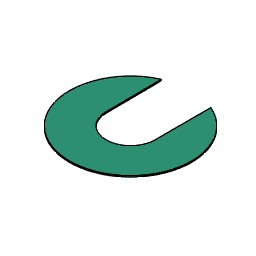
0.2 mm slidable washer - 8mm Shaft v1 (Autodesk Fusion 360 design; units mm, degrees)
Autodesk Fusion 360 part; units mm, degrees
note: some values were not read from the file. Set by a fixed rule: which sketch regions a step uses.
sketch "Sketch1" plane through (0, 0, 0) normal (0, 0, 1) x (1, 0, 0)
  circle A0 centre (0, 0) radius 4
  circle A1 centre (0, 0) radius 10
  line L0 (4, 0) -> (4, 9.1652)
  line L1 (-3.9998, -0.0353) -> (-4.0808, 9.1295)
  dimension "d1" = 8
  dimension "d2" = 20
  constraint coincident A0.centre A1.centre
  constraint coincident A0 L0.start
  constraint coincident A1 L0.end
  constraint tangent A0 L0
  constraint vertical L0
  constraint coincident A0 L1.start
  constraint coincident A1 L1.end
  constraint tangent A0 L1
  measures "d1" diameter of A0
  measures "d2" diameter of A1
extrude "Extrude1" add sketch "Sketch1" along normal blind 0.2 contours A0 A1 L0 L1 picked at (-7.9763, 0.257)
